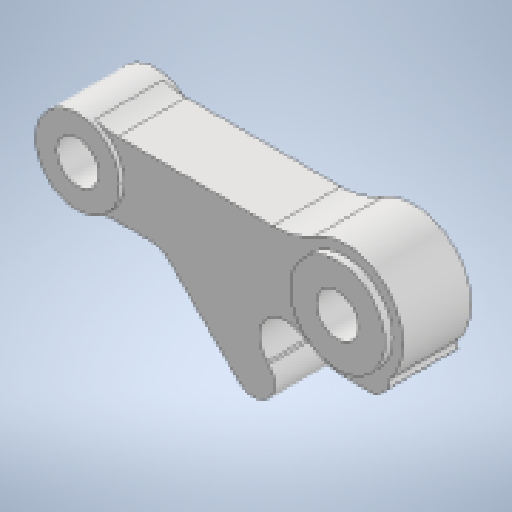
# Autodesk Inventor part: 摇臂
Saved by Autodesk Inventor 2025.1 (Build 291241000, 241)
## iProperties
Created: 2025-08-27
Part Number: 摇臂
Material: 常规
Document SubType Name: Modeling
Designer: Piw
Density: 1 g/cm^3
Appearance: 默认
Author: Piw
Autodesk Inventor part; units mm, degrees
ref_plane "YZ Plane" through (0, 0, 0) normal (1, 0, 0) x (0, 1, 0)
ref_plane "XZ Plane" through (0, 0, 0) normal (0, 1, 0) x (-1, 0, 0)
ref_plane "XY Plane" through (0, 0, 0) normal (0, 0, 1) x (1, 0, 0)
sketch "草图1" plane through (0, 0, 0) normal (0, 0, 1) x (1, 0, 0)
  circle A0 centre (0, 0) radius 4
  dimension "d0" = 8
  constraints: 1 centre point, 1 coincident
  measures "d0" diameter of A0
extrude "拉伸1" add sketch "草图1" along normal blind 7
sketch "草图2" plane through (0, 0, 7) normal (0, 0, 1) x (1, 0, 0)
  circle A0 centre (0, 0) radius 8.5
  dimension "d3" = 17
  constraints: 1 centre point, 1 coincident
  measures "d3" diameter of A0
extrude "拉伸2" add sketch "草图2" along normal blind 1.5
sketch "草图3" plane through (0, 0, 8.5) normal (0, 0, 1) x (1, 0, 0)
  arc A0 (-8.4853, -7) -> (-8.4853, 7) centre (0, 0) ccw
  circle A1 centre (0, 0) radius 4 projected
  line L0 (0, 0) -> (-50, 0) construction
  arc A2 (-42, 0) -> (-46.127, 7) centre (-50, 0) ccw construction
  line L1 (-8.4853, -7) -> (-46.127, -7)
  line L2 (-8.4853, 7) -> (-46.127, 7)
  arc A3 (-11, 0) -> (-8.4853, -7) centre (0, 0) ccw construction
  arc A4 (-8.4853, 7) -> (-11, 0) centre (0, 0) ccw construction
  arc A5 (-46.127, -7) -> (-42, 0) centre (-50, 0) ccw construction
  arc A6 (-46.127, 7) -> (-46.127, -7) centre (-50, 0) ccw
  line L3 (0, 0) -> (8.4853, -8.4853) construction
  line L4 (8.4853, -8.4853) -> (5.9706, -11)
  line L5 (5.9706, -11) -> (0, -11)
  line L6 (8.4853, -8.4853) -> (7.7782, -7.7782)
  dimension "d6" = 22
  dimension "d7" = 50
  dimension "d9" = 7
  dimension "d10" = 8
  dimension "d36" = 12
  dimension "d37" = 135
  dimension "d38" = 135
  constraints: 14 end point, 14 point on circle, 6 centre point, 3 point on line, 2 coincident, 2 symmetric about line, 1 horizontal, 1 parallel, 1 perpendicular, 1 tangent
  measures "d6" diameter of A0
  measures "d7" distance of L0.start L0.end
  measures "d9" distance between parallel lines of L0 L1
  measures "d10" radius of A6
  measures "d36" distance of L0.start L3.end
  measures "d37" angle of L0 L3
  measures "d38" angle of L5 L4
extrude "拉伸3" add sketch "草图3" along normal blind 13 contours L1 A6 L2 A0 | A0 L6 L4 L5 | A1
sketch "草图4" plane through (0, 0, 21.5) normal (0, 0, 1) x (1, 0, 0)
  arc A0 (-8.4853, -7) -> (-8.4853, 7) centre (0, 0) ccw projected
  circle A1 centre (0, 0) radius 9
  dimension "d13" = 18
  constraints: 1 centre point, 1 coincident
  measures "d13" diameter of A1
extrude "拉伸4" add sketch "草图4" along normal blind 1.5
sketch "草图5" plane through (0, 0, 23) normal (0, 0, 1) x (1, 0, 0)
  circle A0 centre (0, 0) radius 4
  dimension "d16" = 8
  constraints: 1 centre point, 1 coincident
  measures "d16" diameter of A0
extrude "拉伸5" add sketch "草图5" along normal blind 7
fillet "圆角1" radius 15 4 edges at (-46.127, 7, 15) (-8.4853, 7, 15) (-8.4853, -7, 15) (-46.127, -7, 15)
sketch "草图6" plane through (0, 0, 21.5) normal (0, 0, 1) x (1, 0, 0)
  arc A0 (-47.6667, 7.6522) -> (-47.6667, -7.6522) centre (-50, 0) ccw projected
  arc A1 (-43.2918, -7) -> (-47.6667, -7.6522) centre (-43.2918, -22) ccw projected
  circle A2 centre (-50, 0) radius 8
  point P0 (0, 0)
  constraints: 1 coincident, 3 other
extrude "拉伸6" add sketch "草图6" along normal blind 0.95
chamfer "倒角1" distance 0.5 angle 45 2 edges at (-4, 0, 30) (-4, 0, 0)
fillet "圆角3" radius 1 2 edges at (7.7782, -7.7782, 15) (5.9706, -11, 15)
sketch "草图10" plane through (0, 0, 30) normal (0, 0, 1) x (1, 0, 0)
  circle A0 centre (0, 0) radius 4 projected
extrude "拉伸10" cut sketch "草图10" against normal blind 30
sketch "草图11" plane through (-50, 0, 22.45) normal (0, 0, 1) x (1, 0, 0)
  circle A0 centre (0, 0) radius 4
  circle A1 centre (0, 0) radius 8 projected
  point P0 (50, 0)
  dimension "d42" = 8
  constraints: 1 centre point, 1 coincident
  measures "d42" diameter of A0
extrude "拉伸11" cut sketch "草图11" against normal blind 30 contours A0
sketch "草图12" plane through (0, 0, 8.5) normal (0, 0, -1) x (-1, 0, 0)
  arc A0 (47.6667, -7.6522) -> (47.6667, 7.6522) centre (50, 0) ccw projected
  circle A1 centre (50, 0) radius 8
  circle A2 centre (50, 0) radius 4 projected
  point P0 (0, 0)
  point P1 (47.6667, -7.6522)
  constraints: 1 coincident, 3 other
extrude "拉伸12" add sketch "草图12" along normal blind 0.95
sketch "草图13" plane through (0, 0, 21.5) normal (0, 0, 1) x (1, 0, 0)
  line L0 (-43.2918, -7) -> (-13.8564, -7) projected
  line L1 (-23.7559, -7) -> (-17.1843, -13.5716)
  arc A0 (-22.8412, -19.2284) -> (-17.1843, -13.5716) centre (-20.0128, -16.4) ccw
  line L2 (-22.8412, -19.2284) -> (-35.0696, -7)
  arc A1 (-17.1843, -13.5716) -> (-22.8412, -19.2284) centre (-20.0128, -16.4) ccw construction
  point P0 (0, 0)
  dimension "d52" = 45
  dimension "d53" = 8
  dimension "d54" = 7
  dimension "d59" = 9.4
  constraints: 4 end point, 4 point on circle, 2 centre point, 2 point on line, 2 tangent, 1 parallel
  measures "d52" angle of L0 L2
  measures "d53" diameter of A0
  measures "d54" distance from line of L1 L0.end
  measures "d59" distance from line of L0 A0.centre
extrude "拉伸13" add sketch "草图13" against normal blind 13
fillet "圆角5" radius 4 1 edges at (-23.7559, -7, 15)
chamfer "倒角2" distance 4 angle 45 1 edges at (-35.0696, -7, 15)
sketch "草图14" plane through (0, 0, 21.5) normal (0, 0, 1) x (1, 0, 0)
  arc A0 (-22.8412, -19.2284) -> (-17.1843, -13.5716) centre (-20.0128, -16.4) ccw projected
  circle A1 centre (-20.0128, -16.4) radius 2.475
  point P0 (0, 0)
  dimension "d64" = 4.95
  constraints: 1 centre point, 1 coincident
  measures "d64" diameter of A1
extrude "拉伸14" cut sketch "草图14" against normal blind 13
